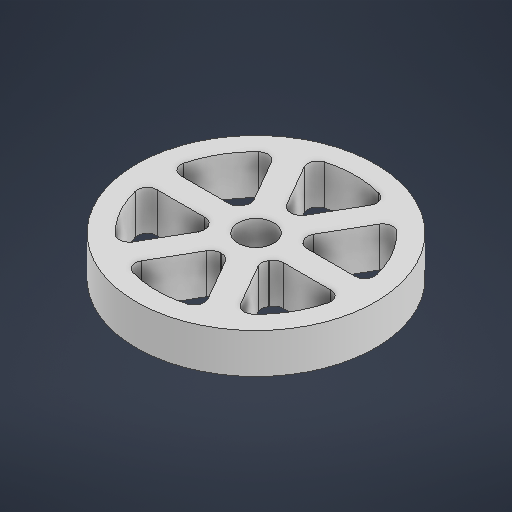
# Autodesk Inventor part: 3in flex
Saved by Autodesk Inventor 2025.2 (Build 292293000, 293)
## iProperties
Created: 2026-01-16
Part Number: 3in flex
Material: Generic
Document SubType Name: Modeling
Designer: cloudy
Density: 1 g/cm^3
Appearance: Default
Author: cloudy
Autodesk Inventor part; units mm, degrees
ref_plane "YZ Plane" through (0, 0, 0) normal (1, 0, 0) x (0, 1, 0)
ref_plane "XZ Plane" through (0, 0, 0) normal (0, 1, 0) x (-1, 0, 0)
ref_plane "XY Plane" through (0, 0, 0) normal (0, 0, 1) x (1, 0, 0)
sketch "Sketch1" plane through (0, 0, 0) normal (0, 1, 0) x (-1, 0, 0)
  circle A0 centre (0, 0) radius 38.1
  circle A1 centre (0, 0) radius 5.715
  line L0 (10.4389, 3.81) -> (31.5206, 3.81)
  line L1 (31.5206, -3.81) -> (10.4389, -3.81)
  line L2 (1.9199, 10.9454) -> (12.4607, 29.2026)
  line L3 (19.0598, 25.3926) -> (8.519, 7.1354)
  line L4 (-8.519, 7.1354) -> (-19.0598, 25.3926)
  line L5 (-12.4607, 29.2026) -> (-1.9199, 10.9454)
  line L6 (-10.4389, -3.81) -> (-31.5206, -3.81)
  line L7 (-31.5206, 3.81) -> (-10.4389, 3.81)
  line L8 (-1.9199, -10.9454) -> (-12.4607, -29.2026)
  line L9 (-19.0598, -25.3926) -> (-8.519, -7.1354)
  line L10 (8.519, -7.1354) -> (19.0598, -25.3926)
  line L11 (12.4607, -29.2026) -> (1.9199, -10.9454)
  arc A2 (10.4389, 3.81) -> (8.519, 7.1354) centre (0, 0) ccw
  arc A3 (1.9199, 10.9454) -> (-1.9199, 10.9454) centre (0, 0) ccw
  arc A4 (-8.519, 7.1354) -> (-10.4389, 3.81) centre (0, 0) ccw
  arc A5 (-10.4389, -3.81) -> (-8.519, -7.1354) centre (0, 0) ccw
  arc A6 (-1.9199, -10.9454) -> (1.9199, -10.9454) centre (0, 0) ccw
  arc A7 (8.519, -7.1354) -> (10.4389, -3.81) centre (0, 0) ccw
  arc A8 (19.0598, -25.3926) -> (31.5206, -3.81) centre (0, 0) ccw
  arc A9 (31.5206, 3.81) -> (19.0598, 25.3926) centre (0, 0) ccw
  arc A10 (12.4607, 29.2026) -> (-12.4607, 29.2026) centre (0, 0) ccw
  arc A11 (-19.0598, 25.3926) -> (-31.5206, 3.81) centre (0, 0) ccw
  arc A12 (-31.5206, -3.81) -> (-19.0598, -25.3926) centre (0, 0) ccw
  arc A13 (-12.4607, -29.2026) -> (12.4607, -29.2026) centre (0, 0) ccw
  dimension "d0" = 76.2
  dimension "d1" = 11.43
  dimension "d4" = 3.81
  dimension "d5" = 3.81
  dimension "d8" = 360
  dimension "d10" = 31.75
  dimension "d11" = 11.1125
  constraints: 24 end point, 24 point on circle, 14 centre point, 4 coincident, 1 horizontal, 1 parallel, 37 other
  measures "d0" diameter of A0
  measures "d1" diameter of A1
  measures "d4" distance from line of point (0, 0) L0
  measures "d5" distance from line of point (0, 0) L1
  measures "d10" radius of A13
  measures "d11" radius of A7
extrude "Extrusion1" add sketch "Sketch1" along normal blind 12.7
fillet "Fillet1" radius 3.175 24 edges at (-19.0598, 6.35, 25.3926) (-12.4607, 6.35, 29.2026) (12.4607, 6.35, 29.2026) (19.0598, 6.35, 25.3926) (31.5206, 6.35, 3.81) (31.5206, 6.35, -3.81) (19.0598, 6.35, -25.3926) (12.4607, 6.35, -29.2026) (-12.4607, 6.35, -29.2026) (-19.0598, 6.35, -25.3926) (-31.5206, 6.35, -3.81) (-31.5206, 6.35, 3.81) (-8.519, 6.35, 7.1354) (-8.519, 6.35, -7.1354) (-10.4389, 6.35, -3.81) (-10.4389, 6.35, 3.81) (-1.9199, 6.35, 10.9454) (1.9199, 6.35, 10.9454) (8.519, 6.35, 7.1354) (10.4389, 6.35, 3.81) (10.4389, 6.35, -3.81) (8.519, 6.35, -7.1354) (1.9199, 6.35, -10.9454) (-1.9199, 6.35, -10.9454)
body "Solid1"
